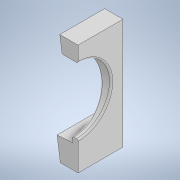
# Autodesk Inventor part: exhastForGasVent02
Saved by Autodesk Inventor 2021.1 (Build 251245000, 245)
## iProperties
Created: 2020-08-27
Part Number: exhastForGasVent02
Material: Generic
Document SubType Name: Modeling
Designer: robst
Density: 1 g/cm^3
Appearance: Default
Author: robst
Autodesk Inventor part; units mm, degrees
ref_plane "YZ Plane" through (0, 0, 0) normal (1, 0, 0) x (0, 1, 0)
ref_plane "XZ Plane" through (0, 0, 0) normal (0, 1, 0) x (-1, 0, 0)
ref_plane "XY Plane" through (0, 0, 0) normal (0, 0, 1) x (1, 0, 0)
sketch "Sketch6" plane through (0, 0, 0) normal (0, 0, 1) x (1, 0, 0)
  line L0 (0, 0) -> (0, 83.82)
  line L1 (0, 83.82) -> (-17.653, 83.82)
  line L2 (-17.653, 83.82) -> (-5.08, 0)
  line L3 (0, 0) -> (0, -22.86)
  line L4 (0, -22.86) -> (-17.091, -22.86)
  line L5 (-23.2881, 0) -> (-5.08, 0) construction
  line L6 (-5.08, 0) -> (-20.32, -1.3333)
  line L7 (-20.32, -1.3333) -> (-17.091, -22.86)
  dimension "d31" = 83.82
  dimension "d32" = 17.653
  dimension "d33" = 22.86
  dimension "d35" = 5
  dimension "d36" = 0
  dimension "d37" = 5.08
  dimension "d47" = 20.32
  constraints: 16 end point, 2 parallel, 2 perpendicular, 2 vertical
  measures "d31" distance of L0.start L0.end
  measures "d32" distance of L0.end L1.end
  measures "d33" distance of L0.start L3.end
  measures "d35" angle of L6 L5
  measures "d36" vertical distance of L2.end L0.start
  measures "d37" distance of L2.end L0.start
  measures "d47" distance from line of L6.end L3
extrude "Extrusion7" add sketch "Sketch6" along normal mid plane 86.36
sketch "Sketch7" plane through (0, -22.86, 43.18) normal (1, 0, 0) x (0, 0, -1)
  line L0 (86.36, 22.86) -> (0, 22.86) projected
  line L1 (0, 106.68) -> (86.36, 106.68) construction
  line L2 (43.18, 106.68) -> (43.18, 22.86) construction
  circle A0 centre (43.18, 59.69) radius 31.75
  dimension "d40" = 63.5
  dimension "d41" = 5.08
  constraints: 2 end point, 1 centre point, 1 midpoint, 1 perpendicular, 1 point on line
  measures "d40" diameter of A0
  measures "d41" distance edge to line of A0 L0
extrude "Extrusion8" cut sketch "Sketch7" against normal through all
sketch "Sketch11" plane through (-17.091, -22.86, -43.18) normal (-0.9889364, -0.1483405, 0) x (0, 0, 1)
  line L0 (43.18, 20.0718) -> (43.18, 0) construction
  line L1 (0, 0) -> (86.36, 0) construction
  line L2 (43.18, 10.0359) -> (86.36, 10.0359) construction
  spline S0 degree 2 poles (51.7003, 11.2824) (51.4336, 11.1738) (50.5806, 10.9663) (50.1656, 10.9663) knots 0 0 0 1 2 2 2
  spline S1 degree 2 poles (50.1656, 10.9663) (49.2073, 10.9663) (48.071, 12.0728) (48.071, 13.0872) knots 0 0 0 1 2 2 2
  spline S2 degree 2 poles (48.071, 13.0872) (48.071, 14.0423) (49.2073, 15.1949) (50.1953, 15.1949) knots 0 0 0 1 2 2 2
  spline S3 degree 2 poles (50.1953, 15.1949) (50.7057, 15.1949) (51.3446, 15.0006) (51.6839, 14.836) knots 0 0 0 1 2 2 2
  line L3 (51.6839, 14.836) -> (51.6839, 13.8809)
  line L4 (51.6839, 13.8809) -> (51.5916, 13.8809)
  spline S4 degree 2 poles (51.5916, 13.8809) (51.5192, 13.9369) (51.2425, 14.1509) (51.1108, 14.2234) knots 0 0 0 1 2 2 2
  spline S5 degree 2 poles (51.1108, 14.2234) (50.9593, 14.3123) (50.5575, 14.4375) (50.3336, 14.4375) knots 0 0 0 1 2 2 2
  spline S6 degree 2 poles (50.3336, 14.4375) (50.0734, 14.4375) (49.642, 14.2728) (49.474, 14.1048) knots 0 0 0 1 2 2 2
  spline S7 degree 2 poles (49.474, 14.1048) (49.3126, 13.9402) (49.1249, 13.4363) (49.1249, 13.1037) knots 0 0 0 1 2 2 2
  spline S8 degree 2 poles (49.1249, 13.1037) (49.1249, 12.3923) (49.8396, 11.7139) (50.4554, 11.7139) knots 0 0 0 1 2 2 2
  spline S9 degree 2 poles (50.4554, 11.7139) (50.5114, 11.7139) (50.6563, 11.7205) (50.7123, 11.7237) knots 0 0 0 1 2 2 2
  line L5 (50.7123, 11.7237) -> (50.7123, 12.524)
  line L6 (50.7123, 12.524) -> (49.9252, 12.524)
  line L7 (49.9252, 12.524) -> (49.9252, 13.2848)
  line L8 (49.9252, 13.2848) -> (51.7003, 13.2848)
  line L9 (51.7003, 13.2848) -> (51.7003, 11.2824)
  spline S10 degree 2 poles (54.1045, 11.3779) (54.0057, 11.2956) (53.8509, 11.1639) (53.7191, 11.098) knots 0 0 0 1 2 2 2
  spline S11 degree 2 poles (53.7191, 11.098) (53.5907, 11.0354) (53.347, 10.9696) (53.1296, 10.9696) knots 0 0 0 1 2 2 2
  spline S12 degree 2 poles (53.1296, 10.9696) (52.7213, 10.9696) (52.1844, 11.5163) (52.1844, 11.9312) knots 0 0 0 1 2 2 2
  spline S13 degree 2 poles (52.1844, 11.9312) (52.1844, 12.2704) (52.4578, 12.692) (52.7147, 12.8138) knots 0 0 0 1 2 2 2
  spline S14 degree 2 poles (52.7147, 12.8138) (52.9748, 12.939) (53.6961, 13.0378) (54.1111, 13.0641) knots 0 0 0 1 2 2 2
  line L10 (54.1111, 13.0641) -> (54.1111, 13.0806)
  spline S15 degree 2 poles (54.1111, 13.0806) (54.1111, 13.3342) (53.7356, 13.5285) (53.3602, 13.5285) knots 0 0 0 1 2 2 2
  spline S16 degree 2 poles (53.3602, 13.5285) (53.1922, 13.5285) (52.7377, 13.4066) (52.5237, 13.3111) knots 0 0 0 1 2 2 2
  line L11 (52.5237, 13.3111) -> (52.4413, 13.3111)
  line L12 (52.4413, 13.3111) -> (52.4413, 14.0521)
  spline S17 degree 2 poles (52.4413, 14.0521) (52.5829, 14.0917) (53.2153, 14.2036) (53.538, 14.2036) knots 0 0 0 1 2 2 2
  spline S18 degree 2 poles (53.538, 14.2036) (54.3284, 14.2036) (55.053, 13.6767) (55.053, 13.1366) knots 0 0 0 1 2 2 2
  line L13 (55.053, 13.1366) -> (55.053, 11.0519)
  line L14 (55.053, 11.0519) -> (54.1045, 11.0519)
  line L15 (54.1045, 11.0519) -> (54.1045, 11.3779)
  line L16 (54.1045, 11.8522) -> (54.1045, 12.4878)
  spline S19 degree 2 poles (54.1045, 12.4878) (53.8608, 12.4647) (53.5611, 12.4285) (53.4162, 12.3758) knots 0 0 0 1 2 2 2
  spline S20 degree 2 poles (53.4162, 12.3758) (53.2877, 12.333) (53.1494, 12.1552) (53.1494, 12.0103) knots 0 0 0 1 2 2 2
  spline S21 degree 2 poles (53.1494, 12.0103) (53.1494, 11.7962) (53.3832, 11.6348) (53.6105, 11.6348) knots 0 0 0 1 2 2 2
  spline S22 degree 2 poles (53.6105, 11.6348) (53.7356, 11.6348) (53.9991, 11.7501) (54.1045, 11.8522) knots 0 0 0 1 2 2 2
  spline S23 degree 2 poles (56.693, 10.9696) (56.3571, 10.9696) (55.7544, 11.1178) (55.5568, 11.2166) knots 0 0 0 1 2 2 2
  line L17 (55.5568, 11.2166) -> (55.5568, 12.0234)
  line L18 (55.5568, 12.0234) -> (55.6359, 12.0234)
  spline S24 degree 2 poles (55.6359, 12.0234) (55.705, 11.9707) (55.8796, 11.8456) (56.0344, 11.7764) knots 0 0 0 1 2 2 2
  spline S25 degree 2 poles (56.0344, 11.7764) (56.1694, 11.7139) (56.502, 11.6249) (56.6996, 11.6249) knots 0 0 0 1 2 2 2
  spline S26 degree 2 poles (56.6996, 11.6249) (56.9005, 11.6249) (57.2101, 11.7501) (57.2101, 11.8851) knots 0 0 0 1 2 2 2
  spline S27 degree 2 poles (57.2101, 11.8851) (57.2101, 11.9905) (57.0685, 12.1025) (56.8643, 12.1486) knots 0 0 0 1 2 2 2
  spline S28 degree 2 poles (56.8643, 12.1486) (56.7556, 12.1782) (56.423, 12.2408) (56.2946, 12.2803) knots 0 0 0 1 2 2 2
  spline S29 degree 2 poles (56.2946, 12.2803) (55.9323, 12.3923) (55.57, 12.8303) (55.57, 13.1893) knots 0 0 0 1 2 2 2
  spline S30 degree 2 poles (55.57, 13.1893) (55.57, 13.3935) (55.7577, 13.7557) (55.9422, 13.8974) knots 0 0 0 1 2 2 2
  spline S31 degree 2 poles (55.9422, 13.8974) (56.1233, 14.0357) (56.6601, 14.2003) (56.9993, 14.2003) knots 0 0 0 1 2 2 2
  spline S32 degree 2 poles (56.9993, 14.2003) (57.3221, 14.2003) (57.8622, 14.0719) (58.0466, 13.983) knots 0 0 0 1 2 2 2
  line L19 (58.0466, 13.983) -> (58.0466, 13.2058)
  line L20 (58.0466, 13.2058) -> (57.9709, 13.2058)
  spline S33 degree 2 poles (57.9709, 13.2058) (57.9215, 13.2453) (57.7074, 13.3737) (57.6086, 13.4198) knots 0 0 0 1 2 2 2
  spline S34 degree 2 poles (57.6086, 13.4198) (57.4867, 13.4725) (57.1903, 13.545) (57.0356, 13.545) knots 0 0 0 1 2 2 2
  spline S35 degree 2 poles (57.0356, 13.545) (56.8281, 13.545) (56.5416, 13.4034) (56.5416, 13.2881) knots 0 0 0 1 2 2 2
  spline S36 degree 2 poles (56.5416, 13.2881) (56.5416, 13.1827) (56.6832, 13.0641) (56.9203, 13.0049) knots 0 0 0 1 2 2 2
  spline S37 degree 2 poles (56.9203, 13.0049) (57.0421, 12.9752) (57.3616, 12.9192) (57.5098, 12.8698) knots 0 0 0 1 2 2 2
  spline S38 degree 2 poles (57.5098, 12.8698) (57.8391, 12.7644) (58.1816, 12.3528) (58.1816, 12.0103) knots 0 0 0 1 2 2 2
  spline S39 degree 2 poles (58.1816, 12.0103) (58.1816, 11.7962) (57.9807, 11.4043) (57.793, 11.2726) knots 0 0 0 1 2 2 2
  spline S40 degree 2 poles (57.793, 11.2726) (57.5987, 11.1276) (57.0652, 10.9696) (56.693, 10.9696) knots 0 0 0 1 2 2 2
  line L21 (63.7211, 15.1159) -> (62.3247, 11.0519)
  line L22 (62.3247, 11.0519) -> (61.2609, 11.0519)
  line L23 (61.2609, 11.0519) -> (59.8645, 15.1159)
  line L24 (59.8645, 15.1159) -> (60.9217, 15.1159)
  line L25 (60.9217, 15.1159) -> (61.8076, 12.3594)
  line L26 (61.8076, 12.3594) -> (62.6902, 15.1159)
  line L27 (62.6902, 15.1159) -> (63.7211, 15.1159)
  spline S41 degree 2 poles (65.7004, 10.9696) (64.8309, 10.9696) (63.9055, 11.7995) (63.9055, 12.5668) knots 0 0 0 1 2 2 2
  spline S42 degree 2 poles (63.9055, 12.5668) (63.9055, 13.3177) (64.7684, 14.2135) (65.5456, 14.2135) knots 0 0 0 1 2 2 2
  spline S43 degree 2 poles (65.5456, 14.2135) (66.2471, 14.2135) (66.9584, 13.4528) (66.9584, 12.748) knots 0 0 0 1 2 2 2
  line L28 (66.9584, 12.748) -> (66.9584, 12.4022)
  line L29 (66.9584, 12.4022) -> (64.8606, 12.4022)
  spline S44 degree 2 poles (64.8606, 12.4022) (64.8737, 12.1881) (65.0285, 11.9049) (65.1537, 11.8193) knots 0 0 0 1 2 2 2
  spline S45 degree 2 poles (65.1537, 11.8193) (65.2755, 11.7336) (65.6049, 11.6612) (65.7992, 11.6612) knots 0 0 0 1 2 2 2
  spline S46 degree 2 poles (65.7992, 11.6612) (65.9638, 11.6612) (66.2866, 11.7336) (66.4216, 11.7962) knots 0 0 0 1 2 2 2
  spline S47 degree 2 poles (66.4216, 11.7962) (66.5402, 11.8456) (66.7378, 11.9675) (66.8004, 12.0136) knots 0 0 0 1 2 2 2
  line L30 (66.8004, 12.0136) -> (66.9024, 12.0136)
  line L31 (66.9024, 12.0136) -> (66.9024, 11.2232)
  spline S48 degree 2 poles (66.9024, 11.2232) (66.7839, 11.177) (66.5929, 11.098) (66.4216, 11.0585) knots 0 0 0 1 2 2 2
  spline S49 degree 2 poles (66.4216, 11.0585) (66.2668, 11.0157) (65.9375, 10.9696) (65.7004, 10.9696) knots 0 0 0 1 2 2 2
  spline S50 degree 2 poles (66.0165, 12.9785) (66.0099, 13.2815) (65.7432, 13.601) (65.4698, 13.601) knots 0 0 0 1 2 2 2
  spline S51 degree 2 poles (65.4698, 13.601) (65.1899, 13.601) (64.8737, 13.265) (64.8573, 12.9785) knots 0 0 0 1 2 2 2
  line L32 (64.8573, 12.9785) -> (66.0165, 12.9785)
  line L33 (70.3177, 11.0519) -> (69.356, 11.0519)
  line L34 (69.356, 11.0519) -> (69.356, 12.5701)
  spline S52 degree 2 poles (69.356, 12.5701) (69.356, 12.7579) (69.3264, 13.1267) (69.2868, 13.2123) knots 0 0 0 1 2 2 2
  spline S53 degree 2 poles (69.2868, 13.2123) (69.2374, 13.3177) (69.053, 13.4066) (68.8949, 13.4066) knots 0 0 0 1 2 2 2
  spline S54 degree 2 poles (68.8949, 13.4066) (68.7797, 13.4066) (68.5392, 13.3177) (68.4042, 13.2222) knots 0 0 0 1 2 2 2
  line L35 (68.4042, 13.2222) -> (68.4042, 11.0519)
  line L36 (68.4042, 11.0519) -> (67.4491, 11.0519)
  line L37 (67.4491, 11.0519) -> (67.4491, 14.118)
  line L38 (67.4491, 14.118) -> (68.4042, 14.118)
  line L39 (68.4042, 14.118) -> (68.4042, 13.7788)
  spline S55 degree 2 poles (68.4042, 13.7788) (68.638, 13.9764) (69.0826, 14.2003) (69.3527, 14.2003) knots 0 0 0 1 2 2 2
  spline S56 degree 2 poles (69.3527, 14.2003) (69.8204, 14.2003) (70.3177, 13.6075) (70.3177, 13.0477) knots 0 0 0 1 2 2 2
  line L40 (70.3177, 13.0477) -> (70.3177, 11.0519)
  spline S57 degree 2 poles (72.1982, 10.9926) (71.6152, 10.9926) (71.0817, 11.4734) (71.0817, 12.0201) knots 0 0 0 1 2 2 2
  line L41 (71.0817, 12.0201) -> (71.0817, 13.4528)
  line L42 (71.0817, 13.4528) -> (70.7162, 13.4528)
  line L43 (70.7162, 13.4528) -> (70.7162, 14.118)
  line L44 (70.7162, 14.118) -> (71.0817, 14.118)
  line L45 (71.0817, 14.118) -> (71.0817, 14.994)
  line L46 (71.0817, 14.994) -> (72.0368, 14.994)
  line L47 (72.0368, 14.994) -> (72.0368, 14.118)
  line L48 (72.0368, 14.118) -> (72.9589, 14.118)
  line L49 (72.9589, 14.118) -> (72.9589, 13.4528)
  line L50 (72.9589, 13.4528) -> (72.0368, 13.4528)
  line L51 (72.0368, 13.4528) -> (72.0368, 12.3627)
  spline S58 degree 2 poles (72.0368, 12.3627) (72.0368, 12.2013) (72.0434, 11.9609) (72.0829, 11.8654) knots 0 0 0 1 2 2 2
  spline S59 degree 2 poles (72.0829, 11.8654) (72.1224, 11.7699) (72.3167, 11.6579) (72.5012, 11.6579) knots 0 0 0 1 2 2 2
  spline S60 degree 2 poles (72.5012, 11.6579) (72.5802, 11.6579) (72.8272, 11.7237) (72.8766, 11.7501) knots 0 0 0 1 2 2 2
  line L52 (72.8766, 11.7501) -> (72.9589, 11.7501)
  line L53 (72.9589, 11.7501) -> (72.9589, 11.0782)
  spline S61 degree 2 poles (72.9589, 11.0782) (72.8041, 11.0387) (72.455, 10.9926) (72.1982, 10.9926) knots 0 0 0 1 2 2 2
  spline S62 degree 2 poles (77.9648, 13.0839) (77.9648, 12.557) (77.7969, 11.7666) (77.6091, 11.4998) knots 0 0 0 1 2 2 2
  spline S63 degree 2 poles (77.6091, 11.4998) (77.4247, 11.2363) (76.8286, 10.9663) (76.4005, 10.9663) knots 0 0 0 1 2 2 2
  spline S64 degree 2 poles (76.4005, 10.9663) (75.9691, 10.9663) (75.3762, 11.2363) (75.1885, 11.5064) knots 0 0 0 1 2 2 2
  spline S65 degree 2 poles (75.1885, 11.5064) (75.0008, 11.7731) (74.8328, 12.557) (74.8328, 13.0839) knots 0 0 0 1 2 2 2
  spline S66 degree 2 poles (74.8328, 13.0839) (74.8328, 13.624) (75.0008, 14.3881) (75.1918, 14.6647) knots 0 0 0 1 2 2 2
  spline S67 degree 2 poles (75.1918, 14.6647) (75.3828, 14.9348) (75.9855, 15.1982) (76.4005, 15.1982) knots 0 0 0 1 2 2 2
  spline S68 degree 2 poles (76.4005, 15.1982) (76.8385, 15.1982) (77.4247, 14.9216) (77.6124, 14.6482) knots 0 0 0 1 2 2 2
  spline S69 degree 2 poles (77.6124, 14.6482) (77.7969, 14.3815) (77.9648, 13.5944) (77.9648, 13.0839) knots 0 0 0 1 2 2 2
  spline S70 degree 2 poles (76.9406, 13.0839) (76.9406, 13.8381) (76.6936, 14.4473) (76.4005, 14.4473) knots 0 0 0 1 2 2 2
  spline S71 degree 2 poles (76.4005, 14.4473) (76.1074, 14.4473) (75.8571, 13.8381) (75.8571, 13.0806) knots 0 0 0 1 2 2 2
  spline S72 degree 2 poles (75.8571, 13.0806) (75.8571, 12.3363) (76.1074, 11.7172) (76.4005, 11.7172) knots 0 0 0 1 2 2 2
  spline S73 degree 2 poles (76.4005, 11.7172) (76.6903, 11.7172) (76.9406, 12.3363) (76.9406, 13.0839) knots 0 0 0 1 2 2 2
  line L54 (81.5776, 11.0519) -> (78.5906, 11.0519)
  line L55 (78.5906, 11.0519) -> (78.5906, 11.7139)
  spline S74 degree 2 poles (78.5906, 11.7139) (78.9693, 12.0169) (79.5753, 12.5504) (79.8025, 12.7908) knots 0 0 0 1 2 2 2
  spline S75 degree 2 poles (79.8025, 12.7908) (80.1022, 13.1037) (80.369, 13.5812) (80.369, 13.8315) knots 0 0 0 1 2 2 2
  spline S76 degree 2 poles (80.369, 13.8315) (80.369, 14.1147) (80.0298, 14.4177) (79.7268, 14.4177) knots 0 0 0 1 2 2 2
  spline S77 degree 2 poles (79.7268, 14.4177) (79.572, 14.4177) (79.2953, 14.342) (79.1537, 14.2827) knots 0 0 0 1 2 2 2
  spline S78 degree 2 poles (79.1537, 14.2827) (79.0154, 14.2201) (78.8178, 14.0884) (78.7684, 14.0554) knots 0 0 0 1 2 2 2
  line L56 (78.7684, 14.0554) -> (78.6894, 14.0554)
  line L57 (78.6894, 14.0554) -> (78.6894, 14.9414)
  spline S79 degree 2 poles (78.6894, 14.9414) (78.8606, 15.0237) (79.5917, 15.1949) (79.931, 15.1949) knots 0 0 0 1 2 2 2
  spline S80 degree 2 poles (79.931, 15.1949) (80.6555, 15.1949) (81.3998, 14.5494) (81.3998, 13.9665) knots 0 0 0 1 2 2 2
  spline S81 degree 2 poles (81.3998, 13.9665) (81.3998, 13.6075) (81.0606, 12.9159) (80.6687, 12.5207) knots 0 0 0 1 2 2 2
  spline S82 degree 2 poles (80.6687, 12.5207) (80.4217, 12.277) (79.9573, 11.8983) (79.8552, 11.8193) knots 0 0 0 1 2 2 2
  line L58 (79.8552, 11.8193) -> (81.5776, 11.8193)
  line L59 (81.5776, 11.8193) -> (81.5776, 11.0519)
  spline S83 degree 2 poles (54.0073, 7.0249) (54.0073, 6.7416) (53.8262, 6.2279) (53.6582, 6.0566) knots 0 0 0 1 2 2 2
  spline S84 degree 2 poles (53.6582, 6.0566) (53.5561, 5.9479) (53.3058, 5.7701) (53.1576, 5.7075) knots 0 0 0 1 2 2 2
  spline S85 degree 2 poles (53.1576, 5.7075) (53.0061, 5.6449) (52.6537, 5.5725) (52.4364, 5.5725) knots 0 0 0 1 2 2 2
  line L60 (52.4364, 5.5725) -> (51.9029, 5.5725)
  line L61 (51.9029, 5.5725) -> (51.9029, 4.242)
  line L62 (51.9029, 4.242) -> (50.8819, 4.242)
  line L63 (50.8819, 4.242) -> (50.8819, 8.306)
  line L64 (50.8819, 8.306) -> (52.4594, 8.306)
  spline S86 degree 2 poles (52.4594, 8.306) (52.8085, 8.306) (53.319, 8.1775) (53.5265, 8.0392) knots 0 0 0 1 2 2 2
  spline S87 degree 2 poles (53.5265, 8.0392) (53.757, 7.8844) (54.0073, 7.3772) (54.0073, 7.0249) knots 0 0 0 1 2 2 2
  spline S88 degree 2 poles (52.96, 6.9985) (52.96, 7.1731) (52.7954, 7.4201) (52.6834, 7.4662) knots 0 0 0 1 2 2 2
  spline S89 degree 2 poles (52.6834, 7.4662) (52.5385, 7.5287) (52.275, 7.5485) (52.0478, 7.5485) knots 0 0 0 1 2 2 2
  line L65 (52.0478, 7.5485) -> (51.9029, 7.5485)
  line L66 (51.9029, 7.5485) -> (51.9029, 6.33)
  line L67 (51.9029, 6.33) -> (51.9753, 6.33)
  spline S90 degree 2 poles (51.9753, 6.33) (52.1169, 6.33) (52.3738, 6.3365) (52.4693, 6.353) knots 0 0 0 1 2 2 2
  spline S91 degree 2 poles (52.4693, 6.353) (52.5517, 6.3662) (52.7328, 6.4452) (52.7822, 6.4946) knots 0 0 0 1 2 2 2
  spline S92 degree 2 poles (52.7822, 6.4946) (52.8876, 6.5934) (52.96, 6.8141) (52.96, 6.9985) knots 0 0 0 1 2 2 2
  line L68 (56.5564, 6.4024) -> (56.4773, 6.4024)
  spline S93 degree 2 poles (56.4773, 6.4024) (56.4213, 6.4222) (56.2139, 6.4419) (56.0887, 6.4419) knots 0 0 0 1 2 2 2
  spline S94 degree 2 poles (56.0887, 6.4419) (55.9405, 6.4419) (55.6079, 6.353) (55.4531, 6.2937) knots 0 0 0 1 2 2 2
  line L69 (55.4531, 6.2937) -> (55.4531, 4.242)
  line L70 (55.4531, 4.242) -> (54.498, 4.242)
  line L71 (54.498, 4.242) -> (54.498, 7.3081)
  line L72 (54.498, 7.3081) -> (55.4531, 7.3081)
  line L73 (55.4531, 7.3081) -> (55.4531, 6.8668)
  spline S95 degree 2 poles (55.4531, 6.8668) (55.519, 6.9261) (55.7495, 7.1105) (55.845, 7.1665) knots 0 0 0 1 2 2 2
  spline S96 degree 2 poles (55.845, 7.1665) (55.9504, 7.229) (56.227, 7.318) (56.3489, 7.318) knots 0 0 0 1 2 2 2
  spline S97 degree 2 poles (56.3489, 7.318) (56.395, 7.318) (56.5103, 7.3114) (56.5564, 7.3081) knots 0 0 0 1 2 2 2
  line L74 (56.5564, 7.3081) -> (56.5564, 6.4024)
  line L75 (57.877, 4.242) -> (56.9219, 4.242)
  line L76 (56.9219, 4.242) -> (56.9219, 7.3081)
  line L77 (56.9219, 7.3081) -> (57.877, 7.3081)
  line L78 (57.877, 7.3081) -> (57.877, 4.242)
  line L79 (57.9066, 7.7461) -> (56.8956, 7.7461)
  line L80 (56.8956, 7.7461) -> (56.8956, 8.4904)
  line L81 (56.8956, 8.4904) -> (57.9066, 8.4904)
  line L82 (57.9066, 8.4904) -> (57.9066, 7.7461)
  line L83 (61.4766, 4.242) -> (60.515, 4.242)
  line L84 (60.515, 4.242) -> (60.515, 5.7602)
  spline S98 degree 2 poles (60.515, 5.7602) (60.515, 5.9479) (60.4853, 6.3168) (60.4458, 6.4024) knots 0 0 0 1 2 2 2
  spline S99 degree 2 poles (60.4458, 6.4024) (60.3964, 6.5078) (60.212, 6.5967) (60.0539, 6.5967) knots 0 0 0 1 2 2 2
  spline S100 degree 2 poles (60.0539, 6.5967) (59.9386, 6.5967) (59.6982, 6.5078) (59.5632, 6.4123) knots 0 0 0 1 2 2 2
  line L85 (59.5632, 6.4123) -> (59.5632, 4.242)
  line L86 (59.5632, 4.242) -> (58.6081, 4.242)
  line L87 (58.6081, 4.242) -> (58.6081, 7.3081)
  line L88 (58.6081, 7.3081) -> (59.5632, 7.3081)
  line L89 (59.5632, 7.3081) -> (59.5632, 6.9689)
  spline S101 degree 2 poles (59.5632, 6.9689) (59.797, 7.1665) (60.2416, 7.3904) (60.5117, 7.3904) knots 0 0 0 1 2 2 2
  spline S102 degree 2 poles (60.5117, 7.3904) (60.9793, 7.3904) (61.4766, 6.7976) (61.4766, 6.2377) knots 0 0 0 1 2 2 2
  line L90 (61.4766, 6.2377) -> (61.4766, 4.242)
  spline S103 degree 2 poles (63.3572, 4.1827) (62.7742, 4.1827) (62.2407, 4.6635) (62.2407, 5.2102) knots 0 0 0 1 2 2 2
  line L91 (62.2407, 5.2102) -> (62.2407, 6.6428)
  line L92 (62.2407, 6.6428) -> (61.8751, 6.6428)
  line L93 (61.8751, 6.6428) -> (61.8751, 7.3081)
  line L94 (61.8751, 7.3081) -> (62.2407, 7.3081)
  line L95 (62.2407, 7.3081) -> (62.2407, 8.1841)
  line L96 (62.2407, 8.1841) -> (63.1958, 8.1841)
  line L97 (63.1958, 8.1841) -> (63.1958, 7.3081)
  line L98 (63.1958, 7.3081) -> (64.1179, 7.3081)
  line L99 (64.1179, 7.3081) -> (64.1179, 6.6428)
  line L100 (64.1179, 6.6428) -> (63.1958, 6.6428)
  line L101 (63.1958, 6.6428) -> (63.1958, 5.5527)
  spline S104 degree 2 poles (63.1958, 5.5527) (63.1958, 5.3914) (63.2024, 5.1509) (63.2419, 5.0554) knots 0 0 0 1 2 2 2
  spline S105 degree 2 poles (63.2419, 5.0554) (63.2814, 4.9599) (63.4757, 4.848) (63.6601, 4.848) knots 0 0 0 1 2 2 2
  spline S106 degree 2 poles (63.6601, 4.848) (63.7392, 4.848) (63.9862, 4.9138) (64.0356, 4.9402) knots 0 0 0 1 2 2 2
  line L102 (64.0356, 4.9402) -> (64.1179, 4.9402)
  line L103 (64.1179, 4.9402) -> (64.1179, 4.2683)
  spline S107 degree 2 poles (64.1179, 4.2683) (63.9631, 4.2288) (63.614, 4.1827) (63.3572, 4.1827) knots 0 0 0 1 2 2 2
  line L104 (69.5915, 8.306) -> (68.1951, 4.242)
  line L105 (68.1951, 4.242) -> (67.1313, 4.242)
  line L106 (67.1313, 4.242) -> (65.735, 8.306)
  line L107 (65.735, 8.306) -> (66.7921, 8.306)
  line L108 (66.7921, 8.306) -> (67.678, 5.5494)
  line L109 (67.678, 5.5494) -> (68.5607, 8.306)
  line L110 (68.5607, 8.306) -> (69.5915, 8.306)
  line L111 (71.742, 5.6581) -> (69.934, 5.6581)
  line L112 (69.934, 5.6581) -> (69.934, 6.4156)
  line L113 (69.934, 6.4156) -> (71.742, 6.4156)
  line L114 (71.742, 6.4156) -> (71.742, 5.6581)
  spline S108 degree 2 poles (75.3911, 6.274) (75.3911, 5.747) (75.2231, 4.9566) (75.0354, 4.6899) knots 0 0 0 1 2 2 2
  spline S109 degree 2 poles (75.0354, 4.6899) (74.851, 4.4264) (74.2549, 4.1563) (73.8267, 4.1563) knots 0 0 0 1 2 2 2
  spline S110 degree 2 poles (73.8267, 4.1563) (73.3953, 4.1563) (72.8025, 4.4264) (72.6148, 4.6965) knots 0 0 0 1 2 2 2
  spline S111 degree 2 poles (72.6148, 4.6965) (72.4271, 4.9632) (72.2591, 5.747) (72.2591, 6.274) knots 0 0 0 1 2 2 2
  spline S112 degree 2 poles (72.2591, 6.274) (72.2591, 6.8141) (72.4271, 7.5781) (72.6181, 7.8548) knots 0 0 0 1 2 2 2
  spline S113 degree 2 poles (72.6181, 7.8548) (72.8091, 8.1248) (73.4118, 8.3883) (73.8267, 8.3883) knots 0 0 0 1 2 2 2
  spline S114 degree 2 poles (73.8267, 8.3883) (74.2647, 8.3883) (74.851, 8.1117) (75.0387, 7.8383) knots 0 0 0 1 2 2 2
  spline S115 degree 2 poles (75.0387, 7.8383) (75.2231, 7.5716) (75.3911, 6.7844) (75.3911, 6.274) knots 0 0 0 1 2 2 2
  spline S116 degree 2 poles (74.3668, 6.274) (74.3668, 7.0282) (74.1198, 7.6374) (73.8267, 7.6374) knots 0 0 0 1 2 2 2
  spline S117 degree 2 poles (73.8267, 7.6374) (73.5336, 7.6374) (73.2833, 7.0282) (73.2833, 6.2707) knots 0 0 0 1 2 2 2
  spline S118 degree 2 poles (73.2833, 6.2707) (73.2833, 5.5264) (73.5336, 4.9072) (73.8267, 4.9072) knots 0 0 0 1 2 2 2
  spline S119 degree 2 poles (73.8267, 4.9072) (74.1165, 4.9072) (74.3668, 5.5264) (74.3668, 6.274) knots 0 0 0 1 2 2 2
  line L115 (79.0039, 4.242) -> (76.0168, 4.242)
  line L116 (76.0168, 4.242) -> (76.0168, 4.9039)
  spline S120 degree 2 poles (76.0168, 4.9039) (76.3955, 5.2069) (77.0015, 5.7405) (77.2288, 5.9809) knots 0 0 0 1 2 2 2
  spline S121 degree 2 poles (77.2288, 5.9809) (77.5285, 6.2937) (77.7952, 6.7713) (77.7952, 7.0216) knots 0 0 0 1 2 2 2
  spline S122 degree 2 poles (77.7952, 7.0216) (77.7952, 7.3048) (77.456, 7.6078) (77.153, 7.6078) knots 0 0 0 1 2 2 2
  spline S123 degree 2 poles (77.153, 7.6078) (76.9982, 7.6078) (76.7216, 7.532) (76.58, 7.4728) knots 0 0 0 1 2 2 2
  spline S124 degree 2 poles (76.58, 7.4728) (76.4416, 7.4102) (76.244, 7.2784) (76.1946, 7.2455) knots 0 0 0 1 2 2 2
  line L117 (76.1946, 7.2455) -> (76.1156, 7.2455)
  line L118 (76.1156, 7.2455) -> (76.1156, 8.1314)
  spline S125 degree 2 poles (76.1156, 8.1314) (76.2869, 8.2138) (77.018, 8.385) (77.3572, 8.385) knots 0 0 0 1 2 2 2
  spline S126 degree 2 poles (77.3572, 8.385) (78.0817, 8.385) (78.826, 7.7395) (78.826, 7.1566) knots 0 0 0 1 2 2 2
  spline S127 degree 2 poles (78.826, 7.1566) (78.826, 6.7976) (78.4868, 6.106) (78.0949, 5.7108) knots 0 0 0 1 2 2 2
  spline S128 degree 2 poles (78.0949, 5.7108) (77.8479, 5.4671) (77.3835, 5.0884) (77.2815, 5.0093) knots 0 0 0 1 2 2 2
  line L119 (77.2815, 5.0093) -> (79.0039, 5.0093)
  line L120 (79.0039, 5.0093) -> (79.0039, 4.242)
  constraints: 4 end point, 2 horizontal, 2 midpoint
extrude "Extrusion11" cut sketch "Sketch11" against normal blind 1.27
fillet "Fillet1" radius 1.5875 2 edges at (0, 36.83, 31.75) (-10.6045, 36.83, 31.75)
sketch "Sketch12" plane through (-17.091, -22.86, -43.18) normal (-0.9889364, -0.1483405, 0) x (0, 0, 1)
  line L0 (43.18, 20.0718) -> (43.18, 0) construction
  line L1 (0, 0) -> (86.36, 0) construction
  line L2 (43.18, 10.0359) -> (0, 10.0359) construction
  line L3 (0, 0) -> (0, 21.7675) construction
  spline S0 degree 2 poles (8.6982, 10.9729) (8.2667, 10.9729) (7.5521, 11.2363) (7.2952, 11.5031) knots 0 0 0 1 2 2 2
  spline S1 degree 2 poles (7.2952, 11.5031) (7.0383, 11.7731) (6.765, 12.5701) (6.765, 13.0872) knots 0 0 0 1 2 2 2
  spline S2 degree 2 poles (6.765, 13.0872) (6.765, 13.5779) (7.0416, 14.3551) (7.2985, 14.6318) knots 0 0 0 1 2 2 2
  spline S3 degree 2 poles (7.2985, 14.6318) (7.5455, 14.8985) (8.27, 15.1884) (8.7015, 15.1884) knots 0 0 0 1 2 2 2
  spline S4 degree 2 poles (8.7015, 15.1884) (8.9089, 15.1884) (9.2844, 15.1291) (9.4556, 15.0764) knots 0 0 0 1 2 2 2
  spline S5 degree 2 poles (9.4556, 15.0764) (9.594, 15.0369) (9.9299, 14.892) (10.032, 14.8393) knots 0 0 0 1 2 2 2
  line L4 (10.032, 14.8393) -> (10.032, 14.1872)
  line L5 (10.032, 14.1872) -> (9.9859, 14.1872)
  spline S6 degree 2 poles (9.9859, 14.1872) (9.8838, 14.2761) (9.6697, 14.4375) (9.4721, 14.5297) knots 0 0 0 1 2 2 2
  spline S7 degree 2 poles (9.4721, 14.5297) (9.3074, 14.612) (8.8826, 14.7207) (8.6389, 14.7207) knots 0 0 0 1 2 2 2
  spline S8 degree 2 poles (8.6389, 14.7207) (8.0527, 14.7207) (7.3281, 13.8381) (7.3281, 13.1037) knots 0 0 0 1 2 2 2
  spline S9 degree 2 poles (7.3281, 13.1037) (7.3281, 12.6953) (7.5191, 12.0827) (7.7003, 11.8719) knots 0 0 0 1 2 2 2
  spline S10 degree 2 poles (7.7003, 11.8719) (7.8748, 11.6612) (8.3688, 11.4405) (8.6784, 11.4405) knots 0 0 0 1 2 2 2
  spline S11 degree 2 poles (8.6784, 11.4405) (8.9056, 11.4405) (9.3601, 11.5064) (9.5149, 11.5722) knots 0 0 0 1 2 2 2
  line L6 (9.5149, 11.5722) -> (9.5149, 12.6228)
  line L7 (9.5149, 12.6228) -> (8.573, 12.6228)
  line L8 (8.573, 12.6228) -> (8.573, 13.0971)
  line L9 (8.573, 13.0971) -> (10.0484, 13.0971)
  line L10 (10.0484, 13.0971) -> (10.0484, 11.322)
  spline S12 degree 2 poles (10.0484, 11.322) (9.9463, 11.2758) (9.5972, 11.1342) (9.449, 11.0914) knots 0 0 0 1 2 2 2
  spline S13 degree 2 poles (9.449, 11.0914) (9.2482, 11.0321) (8.9254, 10.9729) (8.6982, 10.9729) knots 0 0 0 1 2 2 2
  spline S14 degree 2 poles (12.3867, 11.3746) (12.3241, 11.3285) (12.1134, 11.1639) (12.0146, 11.1145) knots 0 0 0 1 2 2 2
  spline S15 degree 2 poles (12.0146, 11.1145) (11.8795, 11.042) (11.626, 10.9663) (11.3954, 10.9663) knots 0 0 0 1 2 2 2
  spline S16 degree 2 poles (11.3954, 10.9663) (11.2077, 10.9663) (10.8685, 11.1079) (10.74, 11.2363) knots 0 0 0 1 2 2 2
  spline S17 degree 2 poles (10.74, 11.2363) (10.6182, 11.3615) (10.47, 11.7303) (10.47, 11.9345) knots 0 0 0 1 2 2 2
  spline S18 degree 2 poles (10.47, 11.9345) (10.47, 12.2507) (10.7367, 12.6986) (11.0266, 12.827) knots 0 0 0 1 2 2 2
  spline S19 degree 2 poles (11.0266, 12.827) (11.2834, 12.9456) (11.9816, 13.0345) (12.3867, 13.0576) knots 0 0 0 1 2 2 2
  line L11 (12.3867, 13.0576) -> (12.3867, 13.1564)
  spline S20 degree 2 poles (12.3867, 13.1564) (12.3867, 13.3342) (12.278, 13.5548) (12.1792, 13.6174) knots 0 0 0 1 2 2 2
  spline S21 degree 2 poles (12.1792, 13.6174) (12.0804, 13.68) (11.7972, 13.7195) (11.6457, 13.7195) knots 0 0 0 1 2 2 2
  spline S22 degree 2 poles (11.6457, 13.7195) (11.4679, 13.7195) (10.987, 13.6141) (10.7466, 13.512) knots 0 0 0 1 2 2 2
  line L12 (10.7466, 13.512) -> (10.717, 13.512)
  line L13 (10.717, 13.512) -> (10.717, 14.0357)
  spline S23 degree 2 poles (10.717, 14.0357) (10.8586, 14.0752) (11.3888, 14.174) (11.649, 14.174) knots 0 0 0 1 2 2 2
  spline S24 degree 2 poles (11.649, 14.174) (11.9652, 14.174) (12.3966, 14.0752) (12.5679, 13.9468) knots 0 0 0 1 2 2 2
  spline S25 degree 2 poles (12.5679, 13.9468) (12.7358, 13.8216) (12.9005, 13.4231) (12.9005, 13.1366) knots 0 0 0 1 2 2 2
  line L14 (12.9005, 13.1366) -> (12.9005, 11.0519)
  line L15 (12.9005, 11.0519) -> (12.3867, 11.0519)
  line L16 (12.3867, 11.0519) -> (12.3867, 11.3746)
  line L17 (12.3867, 11.8028) -> (12.3867, 12.6492)
  spline S26 degree 2 poles (12.3867, 12.6492) (12.2023, 12.6327) (11.6457, 12.5767) (11.4712, 12.524) knots 0 0 0 1 2 2 2
  spline S27 degree 2 poles (11.4712, 12.524) (11.267, 12.4615) (11.0002, 12.2013) (11.0002, 11.9707) knots 0 0 0 1 2 2 2
  spline S28 degree 2 poles (11.0002, 11.9707) (11.0002, 11.7073) (11.2966, 11.4405) (11.5798, 11.4405) knots 0 0 0 1 2 2 2
  spline S29 degree 2 poles (11.5798, 11.4405) (11.8203, 11.4405) (12.2155, 11.648) (12.3867, 11.8028) knots 0 0 0 1 2 2 2
  spline S30 degree 2 poles (14.4451, 10.9794) (14.1388, 10.9794) (13.6086, 11.1441) (13.434, 11.2363) knots 0 0 0 1 2 2 2
  line L18 (13.434, 11.2363) -> (13.434, 11.8127)
  line L19 (13.434, 11.8127) -> (13.4604, 11.8127)
  spline S31 degree 2 poles (13.4604, 11.8127) (13.5262, 11.76) (13.7041, 11.6348) (13.8523, 11.5657) knots 0 0 0 1 2 2 2
  spline S32 degree 2 poles (13.8523, 11.5657) (13.9807, 11.5031) (14.2969, 11.4109) (14.4648, 11.4109) knots 0 0 0 1 2 2 2
  spline S33 degree 2 poles (14.4648, 11.4109) (14.5867, 11.4109) (14.8666, 11.4669) (14.9325, 11.513) knots 0 0 0 1 2 2 2
  spline S34 degree 2 poles (14.9325, 11.513) (15.028, 11.5755) (15.1136, 11.7172) (15.1136, 11.8621) knots 0 0 0 1 2 2 2
  spline S35 degree 2 poles (15.1136, 11.8621) (15.1136, 12.0432) (14.916, 12.2309) (14.6624, 12.2935) knots 0 0 0 1 2 2 2
  spline S36 degree 2 poles (14.6624, 12.2935) (14.5636, 12.3165) (14.2475, 12.3824) (14.1124, 12.4186) knots 0 0 0 1 2 2 2
  spline S37 degree 2 poles (14.1124, 12.4186) (13.7633, 12.5207) (13.4472, 12.9423) (13.4472, 13.242) knots 0 0 0 1 2 2 2
  spline S38 degree 2 poles (13.4472, 13.242) (13.4472, 13.6569) (14.0696, 14.174) (14.5834, 14.174) knots 0 0 0 1 2 2 2
  spline S39 degree 2 poles (14.5834, 14.174) (14.837, 14.174) (15.3507, 14.0489) (15.5253, 13.9533) knots 0 0 0 1 2 2 2
  line L20 (15.5253, 13.9533) -> (15.5253, 13.4034)
  line L21 (15.5253, 13.4034) -> (15.4989, 13.4034)
  spline S40 degree 2 poles (15.4989, 13.4034) (15.3013, 13.5614) (14.8205, 13.7426) (14.5735, 13.7426) knots 0 0 0 1 2 2 2
  spline S41 degree 2 poles (14.5735, 13.7426) (14.3199, 13.7426) (13.9708, 13.5285) (13.9708, 13.3144) knots 0 0 0 1 2 2 2
  spline S42 degree 2 poles (13.9708, 13.3144) (13.9708, 13.1201) (14.1783, 12.9324) (14.4088, 12.8731) knots 0 0 0 1 2 2 2
  spline S43 degree 2 poles (14.4088, 12.8731) (14.5208, 12.8435) (14.804, 12.7842) (14.9588, 12.748) knots 0 0 0 1 2 2 2
  spline S44 degree 2 poles (14.9588, 12.748) (15.2948, 12.6623) (15.6373, 12.2704) (15.6373, 11.9312) knots 0 0 0 1 2 2 2
  spline S45 degree 2 poles (15.6373, 11.9312) (15.6373, 11.7336) (15.4825, 11.3845) (15.331, 11.2561) knots 0 0 0 1 2 2 2
  spline S46 degree 2 poles (15.331, 11.2561) (15.1696, 11.1211) (14.7579, 10.9794) (14.4451, 10.9794) knots 0 0 0 1 2 2 2
  line L22 (20.8473, 15.1159) -> (19.4477, 11.0519)
  line L23 (19.4477, 11.0519) -> (18.8647, 11.0519)
  line L24 (18.8647, 11.0519) -> (17.4651, 15.1159)
  line L25 (17.4651, 15.1159) -> (18.0447, 15.1159)
  line L26 (18.0447, 15.1159) -> (19.171, 11.7402)
  line L27 (19.171, 11.7402) -> (20.2974, 15.1159)
  line L28 (20.2974, 15.1159) -> (20.8473, 15.1159)
  spline S47 degree 2 poles (22.5665, 10.9827) (21.8354, 10.9827) (21.0318, 11.8028) (21.0318, 12.5603) knots 0 0 0 1 2 2 2
  spline S48 degree 2 poles (21.0318, 12.5603) (21.0318, 13.3046) (21.8123, 14.1872) (22.4413, 14.1872) knots 0 0 0 1 2 2 2
  spline S49 degree 2 poles (22.4413, 14.1872) (22.7246, 14.1872) (23.1626, 14.0225) (23.324, 13.848) knots 0 0 0 1 2 2 2
  spline S50 degree 2 poles (23.324, 13.848) (23.4886, 13.6734) (23.6632, 13.1695) (23.6632, 12.804) knots 0 0 0 1 2 2 2
  line L29 (23.6632, 12.804) -> (23.6632, 12.524)
  line L30 (23.6632, 12.524) -> (21.5521, 12.524)
  spline S51 degree 2 poles (21.5521, 12.524) (21.5521, 11.9938) (22.0856, 11.4306) (22.5599, 11.4306) knots 0 0 0 1 2 2 2
  spline S52 degree 2 poles (22.5599, 11.4306) (22.7279, 11.4306) (23.0539, 11.5064) (23.1856, 11.5657) knots 0 0 0 1 2 2 2
  spline S53 degree 2 poles (23.1856, 11.5657) (23.324, 11.6315) (23.515, 11.7468) (23.5775, 11.7995) knots 0 0 0 1 2 2 2
  line L31 (23.5775, 11.7995) -> (23.6072, 11.7995)
  line L32 (23.6072, 11.7995) -> (23.6072, 11.2396)
  spline S54 degree 2 poles (23.6072, 11.2396) (23.5183, 11.2034) (23.2482, 11.098) (23.1428, 11.0684) knots 0 0 0 1 2 2 2
  spline S55 degree 2 poles (23.1428, 11.0684) (22.9946, 11.0256) (22.7509, 10.9827) (22.5665, 10.9827) knots 0 0 0 1 2 2 2
  spline S56 degree 2 poles (23.1626, 12.9159) (23.156, 13.1234) (23.0704, 13.4264) (22.988, 13.5285) knots 0 0 0 1 2 2 2
  spline S57 degree 2 poles (22.988, 13.5285) (22.8991, 13.6438) (22.6192, 13.7656) (22.4117, 13.7656) knots 0 0 0 1 2 2 2
  spline S58 degree 2 poles (22.4117, 13.7656) (22.2075, 13.7656) (21.921, 13.6438) (21.8024, 13.5252) knots 0 0 0 1 2 2 2
  spline S59 degree 2 poles (21.8024, 13.5252) (21.6872, 13.4034) (21.5686, 13.1102) (21.5521, 12.9159) knots 0 0 0 1 2 2 2
  line L33 (21.5521, 12.9159) -> (23.1626, 12.9159)
  line L34 (26.5778, 11.0519) -> (26.064, 11.0519)
  line L35 (26.064, 11.0519) -> (26.064, 12.7908)
  spline S60 degree 2 poles (26.064, 12.7908) (26.064, 13.0016) (26.0245, 13.3638) (25.9652, 13.4725) knots 0 0 0 1 2 2 2
  spline S61 degree 2 poles (25.9652, 13.4725) (25.9026, 13.5878) (25.6787, 13.6998) (25.4877, 13.6998) knots 0 0 0 1 2 2 2
  spline S62 degree 2 poles (25.4877, 13.6998) (25.2967, 13.6998) (24.8916, 13.4956) (24.6973, 13.3309) knots 0 0 0 1 2 2 2
  line L36 (24.6973, 13.3309) -> (24.6973, 11.0519)
  line L37 (24.6973, 11.0519) -> (24.1835, 11.0519)
  line L38 (24.1835, 11.0519) -> (24.1835, 14.1015)
  line L39 (24.1835, 14.1015) -> (24.6973, 14.1015)
  line L40 (24.6973, 14.1015) -> (24.6973, 13.7623)
  spline S63 degree 2 poles (24.6973, 13.7623) (24.9278, 13.9698) (25.3724, 14.1872) (25.6227, 14.1872) knots 0 0 0 1 2 2 2
  spline S64 degree 2 poles (25.6227, 14.1872) (26.0706, 14.1872) (26.5778, 13.5944) (26.5778, 13.0312) knots 0 0 0 1 2 2 2
  line L41 (26.5778, 13.0312) -> (26.5778, 11.0519)
  spline S65 degree 2 poles (28.2212, 10.9926) (27.8029, 10.9926) (27.332, 11.4702) (27.332, 11.9872) knots 0 0 0 1 2 2 2
  line L42 (27.332, 11.9872) -> (27.332, 13.6767)
  line L43 (27.332, 13.6767) -> (26.9862, 13.6767)
  line L44 (26.9862, 13.6767) -> (26.9862, 14.1015)
  line L45 (26.9862, 14.1015) -> (27.332, 14.1015)
  line L46 (27.332, 14.1015) -> (27.332, 14.9776)
  line L47 (27.332, 14.9776) -> (27.8457, 14.9776)
  line L48 (27.8457, 14.9776) -> (27.8457, 14.1015)
  line L49 (27.8457, 14.1015) -> (28.7909, 14.1015)
  line L50 (28.7909, 14.1015) -> (28.7909, 13.6767)
  line L51 (28.7909, 13.6767) -> (27.8457, 13.6767)
  line L52 (27.8457, 13.6767) -> (27.8457, 12.2243)
  spline S66 degree 2 poles (27.8457, 12.2243) (27.8457, 11.9938) (27.8622, 11.7402) (27.9182, 11.6315) knots 0 0 0 1 2 2 2
  spline S67 degree 2 poles (27.9182, 11.6315) (27.9643, 11.536) (28.1718, 11.4405) (28.3496, 11.4405) knots 0 0 0 1 2 2 2
  spline S68 degree 2 poles (28.3496, 11.4405) (28.4748, 11.4405) (28.7086, 11.5163) (28.7613, 11.5393) knots 0 0 0 1 2 2 2
  line L53 (28.7613, 11.5393) -> (28.7909, 11.5393)
  line L54 (28.7909, 11.5393) -> (28.7909, 11.0782)
  spline S69 degree 2 poles (28.7909, 11.0782) (28.646, 11.0387) (28.3496, 10.9926) (28.2212, 10.9926) knots 0 0 0 1 2 2 2
  spline S70 degree 2 poles (33.3687, 13.0839) (33.3687, 11.9905) (32.7331, 10.9663) (32.0711, 10.9663) knots 0 0 0 1 2 2 2
  spline S71 degree 2 poles (32.0711, 10.9663) (31.3993, 10.9663) (30.7702, 12.0103) (30.7702, 13.0806) knots 0 0 0 1 2 2 2
  spline S72 degree 2 poles (30.7702, 13.0806) (30.7702, 14.1806) (31.4058, 15.1982) (32.0711, 15.1982) knots 0 0 0 1 2 2 2
  spline S73 degree 2 poles (32.0711, 15.1982) (32.7397, 15.1982) (33.3687, 14.1444) (33.3687, 13.0839) knots 0 0 0 1 2 2 2
  spline S74 degree 2 poles (32.6705, 11.8456) (32.7495, 12.0465) (32.8154, 12.6656) (32.8154, 13.0839) knots 0 0 0 1 2 2 2
  spline S75 degree 2 poles (32.8154, 13.0839) (32.8154, 13.5022) (32.7495, 14.118) (32.6672, 14.3255) knots 0 0 0 1 2 2 2
  spline S76 degree 2 poles (32.6672, 14.3255) (32.5849, 14.533) (32.2983, 14.747) (32.0711, 14.747) knots 0 0 0 1 2 2 2
  spline S77 degree 2 poles (32.0711, 14.747) (31.8439, 14.747) (31.5508, 14.533) (31.4651, 14.3189) knots 0 0 0 1 2 2 2
  spline S78 degree 2 poles (31.4651, 14.3189) (31.3828, 14.1114) (31.3235, 13.4791) (31.3235, 13.0806) knots 0 0 0 1 2 2 2
  spline S79 degree 2 poles (31.3235, 13.0806) (31.3235, 12.6525) (31.3762, 12.0794) (31.4618, 11.8555) knots 0 0 0 1 2 2 2
  spline S80 degree 2 poles (31.4618, 11.8555) (31.5409, 11.6447) (31.834, 11.4175) (32.0711, 11.4175) knots 0 0 0 1 2 2 2
  spline S81 degree 2 poles (32.0711, 11.4175) (32.295, 11.4175) (32.5882, 11.6315) (32.6705, 11.8456) knots 0 0 0 1 2 2 2
  line L55 (36.3953, 11.0519) -> (33.889, 11.0519)
  line L56 (33.889, 11.0519) -> (33.889, 11.6282)
  spline S82 degree 2 poles (33.889, 11.6282) (34.1591, 11.8818) (34.6399, 12.3528) (34.8705, 12.6064) knots 0 0 0 1 2 2 2
  spline S83 degree 2 poles (34.8705, 12.6064) (35.3348, 13.1168) (35.674, 13.7294) (35.674, 14.0554) knots 0 0 0 1 2 2 2
  spline S84 degree 2 poles (35.674, 14.0554) (35.674, 14.2267) (35.5686, 14.4836) (35.4731, 14.5659) knots 0 0 0 1 2 2 2
  spline S85 degree 2 poles (35.4731, 14.5659) (35.3776, 14.6482) (35.1273, 14.7306) (34.9758, 14.7306) knots 0 0 0 1 2 2 2
  spline S86 degree 2 poles (34.9758, 14.7306) (34.8309, 14.7306) (34.5345, 14.6581) (34.3995, 14.6021) knots 0 0 0 1 2 2 2
  spline S87 degree 2 poles (34.3995, 14.6021) (34.2842, 14.556) (34.0702, 14.4243) (34.0043, 14.3782) knots 0 0 0 1 2 2 2
  line L57 (34.0043, 14.3782) -> (33.9747, 14.3782)
  line L58 (33.9747, 14.3782) -> (33.9747, 14.9578)
  spline S88 degree 2 poles (33.9747, 14.9578) (34.1426, 15.0402) (34.7453, 15.2015) (35.0154, 15.2015) knots 0 0 0 1 2 2 2
  spline S89 degree 2 poles (35.0154, 15.2015) (35.5851, 15.2015) (36.2273, 14.5988) (36.2273, 14.0851) knots 0 0 0 1 2 2 2
  spline S90 degree 2 poles (36.2273, 14.0851) (36.2273, 13.8447) (36.1153, 13.4429) (36.0165, 13.2716) knots 0 0 0 1 2 2 2
  spline S91 degree 2 poles (36.0165, 13.2716) (35.9177, 13.0938) (35.6312, 12.7447) (35.4731, 12.5767) knots 0 0 0 1 2 2 2
  spline S92 degree 2 poles (35.4731, 12.5767) (35.2163, 12.2968) (34.5872, 11.6974) (34.3995, 11.5228) knots 0 0 0 1 2 2 2
  line L59 (34.3995, 11.5228) -> (36.3953, 11.5228)
  line L60 (36.3953, 11.5228) -> (36.3953, 11.0519)
  spline S93 degree 2 poles (12.2846, 7.1796) (12.2846, 6.9162) (12.0969, 6.4419) (11.9289, 6.2773) knots 0 0 0 1 2 2 2
  spline S94 degree 2 poles (11.9289, 6.2773) (11.7182, 6.0698) (11.1484, 5.8557) (10.7137, 5.8557) knots 0 0 0 1 2 2 2
  line L61 (10.7137, 5.8557) -> (10.2559, 5.8557)
  line L62 (10.2559, 5.8557) -> (10.2559, 4.3408)
  line L63 (10.2559, 4.3408) -> (9.7158, 4.3408)
  line L64 (9.7158, 4.3408) -> (9.7158, 8.4048)
  line L65 (9.7158, 8.4048) -> (10.7367, 8.4048)
  spline S95 degree 2 poles (10.7367, 8.4048) (11.099, 8.4048) (11.6062, 8.2862) (11.8005, 8.1512) knots 0 0 0 1 2 2 2
  spline S96 degree 2 poles (11.8005, 8.1512) (12.0277, 7.9964) (12.2846, 7.5189) (12.2846, 7.1796) knots 0 0 0 1 2 2 2
  spline S97 degree 2 poles (11.7215, 7.1632) (11.7215, 7.374) (11.5766, 7.6835) (11.4284, 7.7823) knots 0 0 0 1 2 2 2
  spline S98 degree 2 poles (11.4284, 7.7823) (11.2999, 7.868) (10.9574, 7.9371) (10.7038, 7.9371) knots 0 0 0 1 2 2 2
  line L66 (10.7038, 7.9371) -> (10.2559, 7.9371)
  line L67 (10.2559, 7.9371) -> (10.2559, 6.3168)
  line L68 (10.2559, 6.3168) -> (10.6248, 6.3168)
  spline S99 degree 2 poles (10.6248, 6.3168) (10.9541, 6.3168) (11.3592, 6.4222) (11.4909, 6.5605) knots 0 0 0 1 2 2 2
  spline S100 degree 2 poles (11.4909, 6.5605) (11.6128, 6.6824) (11.7215, 6.9689) (11.7215, 7.1632) knots 0 0 0 1 2 2 2
  line L69 (14.3759, 6.8404) -> (14.3496, 6.8404)
  spline S101 degree 2 poles (14.3496, 6.8404) (14.2903, 6.8569) (14.1618, 6.8635) (14.0729, 6.8635) knots 0 0 0 1 2 2 2
  spline S102 degree 2 poles (14.0729, 6.8635) (13.8654, 6.8635) (13.4571, 6.6824) (13.2726, 6.5045) knots 0 0 0 1 2 2 2
  line L70 (13.2726, 6.5045) -> (13.2726, 4.3408)
  line L71 (13.2726, 4.3408) -> (12.7589, 4.3408)
  line L72 (12.7589, 4.3408) -> (12.7589, 7.3904)
  line L73 (12.7589, 7.3904) -> (13.2726, 7.3904)
  line L74 (13.2726, 7.3904) -> (13.2726, 6.9359)
  spline S103 degree 2 poles (13.2726, 6.9359) (13.5526, 7.1862) (13.9708, 7.3904) (14.1684, 7.3904) knots 0 0 0 1 2 2 2
  spline S104 degree 2 poles (14.1684, 7.3904) (14.2475, 7.3904) (14.3265, 7.3838) (14.3759, 7.374) knots 0 0 0 1 2 2 2
  line L75 (14.3759, 7.374) -> (14.3759, 6.8404)
  line L76 (15.298, 4.3408) -> (14.7843, 4.3408)
  line L77 (14.7843, 4.3408) -> (14.7843, 7.3904)
  line L78 (14.7843, 7.3904) -> (15.298, 7.3904)
  line L79 (15.298, 7.3904) -> (15.298, 4.3408)
  line L80 (15.3343, 7.8976) -> (14.7513, 7.8976)
  line L81 (14.7513, 7.8976) -> (14.7513, 8.4311)
  line L82 (14.7513, 8.4311) -> (15.3343, 8.4311)
  line L83 (15.3343, 8.4311) -> (15.3343, 7.8976)
  line L84 (18.4465, 4.3408) -> (17.9327, 4.3408)
  line L85 (17.9327, 4.3408) -> (17.9327, 6.0797)
  spline S105 degree 2 poles (17.9327, 6.0797) (17.9327, 6.2904) (17.8932, 6.6527) (17.8339, 6.7614) knots 0 0 0 1 2 2 2
  spline S106 degree 2 poles (17.8339, 6.7614) (17.7714, 6.8767) (17.5474, 6.9886) (17.3564, 6.9886) knots 0 0 0 1 2 2 2
  spline S107 degree 2 poles (17.3564, 6.9886) (17.1654, 6.9886) (16.7603, 6.7844) (16.566, 6.6198) knots 0 0 0 1 2 2 2
  line L86 (16.566, 6.6198) -> (16.566, 4.3408)
  line L87 (16.566, 4.3408) -> (16.0522, 4.3408)
  line L88 (16.0522, 4.3408) -> (16.0522, 7.3904)
  line L89 (16.0522, 7.3904) -> (16.566, 7.3904)
  line L90 (16.566, 7.3904) -> (16.566, 7.0512)
  spline S108 degree 2 poles (16.566, 7.0512) (16.7965, 7.2587) (17.2411, 7.476) (17.4914, 7.476) knots 0 0 0 1 2 2 2
  spline S109 degree 2 poles (17.4914, 7.476) (17.9393, 7.476) (18.4465, 6.8832) (18.4465, 6.3201) knots 0 0 0 1 2 2 2
  line L91 (18.4465, 6.3201) -> (18.4465, 4.3408)
  spline S110 degree 2 poles (20.0899, 4.2815) (19.6716, 4.2815) (19.2007, 4.759) (19.2007, 5.2761) knots 0 0 0 1 2 2 2
  line L92 (19.2007, 5.2761) -> (19.2007, 6.9656)
  line L93 (19.2007, 6.9656) -> (18.8549, 6.9656)
  line L94 (18.8549, 6.9656) -> (18.8549, 7.3904)
  line L95 (18.8549, 7.3904) -> (19.2007, 7.3904)
  line L96 (19.2007, 7.3904) -> (19.2007, 8.2665)
  line L97 (19.2007, 8.2665) -> (19.7144, 8.2665)
  line L98 (19.7144, 8.2665) -> (19.7144, 7.3904)
  line L99 (19.7144, 7.3904) -> (20.6596, 7.3904)
  line L100 (20.6596, 7.3904) -> (20.6596, 6.9656)
  line L101 (20.6596, 6.9656) -> (19.7144, 6.9656)
  line L102 (19.7144, 6.9656) -> (19.7144, 5.5132)
  spline S111 degree 2 poles (19.7144, 5.5132) (19.7144, 5.2827) (19.7309, 5.0291) (19.7869, 4.9204) knots 0 0 0 1 2 2 2
  spline S112 degree 2 poles (19.7869, 4.9204) (19.833, 4.8249) (20.0405, 4.7294) (20.2183, 4.7294) knots 0 0 0 1 2 2 2
  spline S113 degree 2 poles (20.2183, 4.7294) (20.3435, 4.7294) (20.5773, 4.8051) (20.63, 4.8282) knots 0 0 0 1 2 2 2
  line L103 (20.63, 4.8282) -> (20.6596, 4.8282)
  line L104 (20.6596, 4.8282) -> (20.6596, 4.3671)
  spline S114 degree 2 poles (20.6596, 4.3671) (20.5147, 4.3276) (20.2183, 4.2815) (20.0899, 4.2815) knots 0 0 0 1 2 2 2
  line L105 (25.7709, 8.4048) -> (24.3712, 4.3408)
  line L106 (24.3712, 4.3408) -> (23.7883, 4.3408)
  line L107 (23.7883, 4.3408) -> (22.3886, 8.4048)
  line L108 (22.3886, 8.4048) -> (22.9683, 8.4048)
  line L109 (22.9683, 8.4048) -> (24.0946, 5.0291)
  line L110 (24.0946, 5.0291) -> (25.2209, 8.4048)
  line L111 (25.2209, 8.4048) -> (25.7709, 8.4048)
  line L112 (27.579, 5.8722) -> (26.041, 5.8722)
  line L113 (26.041, 5.8722) -> (26.041, 6.3662)
  line L114 (26.041, 6.3662) -> (27.579, 6.3662)
  line L115 (27.579, 6.3662) -> (27.579, 5.8722)
  spline S115 degree 2 poles (30.6484, 6.3728) (30.6484, 5.2794) (30.0128, 4.2551) (29.3508, 4.2551) knots 0 0 0 1 2 2 2
  spline S116 degree 2 poles (29.3508, 4.2551) (28.6789, 4.2551) (28.0499, 5.2991) (28.0499, 6.3695) knots 0 0 0 1 2 2 2
  spline S117 degree 2 poles (28.0499, 6.3695) (28.0499, 7.4695) (28.6855, 8.4871) (29.3508, 8.4871) knots 0 0 0 1 2 2 2
  spline S118 degree 2 poles (29.3508, 8.4871) (30.0193, 8.4871) (30.6484, 7.4332) (30.6484, 6.3728) knots 0 0 0 1 2 2 2
  spline S119 degree 2 poles (29.9502, 5.1345) (30.0292, 5.3354) (30.0951, 5.9545) (30.0951, 6.3728) knots 0 0 0 1 2 2 2
  spline S120 degree 2 poles (30.0951, 6.3728) (30.0951, 6.791) (30.0292, 7.4069) (29.9469, 7.6144) knots 0 0 0 1 2 2 2
  spline S121 degree 2 poles (29.9469, 7.6144) (29.8646, 7.8219) (29.578, 8.0359) (29.3508, 8.0359) knots 0 0 0 1 2 2 2
  spline S122 degree 2 poles (29.3508, 8.0359) (29.1235, 8.0359) (28.8304, 7.8219) (28.7448, 7.6078) knots 0 0 0 1 2 2 2
  spline S123 degree 2 poles (28.7448, 7.6078) (28.6625, 7.4003) (28.6032, 6.768) (28.6032, 6.3695) knots 0 0 0 1 2 2 2
  spline S124 degree 2 poles (28.6032, 6.3695) (28.6032, 5.9413) (28.6559, 5.3683) (28.7415, 5.1444) knots 0 0 0 1 2 2 2
  spline S125 degree 2 poles (28.7415, 5.1444) (28.8206, 4.9336) (29.1137, 4.7063) (29.3508, 4.7063) knots 0 0 0 1 2 2 2
  spline S126 degree 2 poles (29.3508, 4.7063) (29.5747, 4.7063) (29.8678, 4.9204) (29.9502, 5.1345) knots 0 0 0 1 2 2 2
  line L116 (33.675, 4.3408) -> (31.1687, 4.3408)
  line L117 (31.1687, 4.3408) -> (31.1687, 4.9171)
  spline S127 degree 2 poles (31.1687, 4.9171) (31.4388, 5.1707) (31.9196, 5.6417) (32.1501, 5.8952) knots 0 0 0 1 2 2 2
  spline S128 degree 2 poles (32.1501, 5.8952) (32.6145, 6.4057) (32.9537, 7.0183) (32.9537, 7.3443) knots 0 0 0 1 2 2 2
  spline S129 degree 2 poles (32.9537, 7.3443) (32.9537, 7.5156) (32.8483, 7.7725) (32.7528, 7.8548) knots 0 0 0 1 2 2 2
  spline S130 degree 2 poles (32.7528, 7.8548) (32.6573, 7.9371) (32.407, 8.0195) (32.2555, 8.0195) knots 0 0 0 1 2 2 2
  spline S131 degree 2 poles (32.2555, 8.0195) (32.1106, 8.0195) (31.8142, 7.947) (31.6792, 7.891) knots 0 0 0 1 2 2 2
  spline S132 degree 2 poles (31.6792, 7.891) (31.5639, 7.8449) (31.3499, 7.7132) (31.284, 7.6671) knots 0 0 0 1 2 2 2
  line L118 (31.284, 7.6671) -> (31.2544, 7.6671)
  line L119 (31.2544, 7.6671) -> (31.2544, 8.2467)
  spline S133 degree 2 poles (31.2544, 8.2467) (31.4223, 8.329) (32.025, 8.4904) (32.2951, 8.4904) knots 0 0 0 1 2 2 2
  spline S134 degree 2 poles (32.2951, 8.4904) (32.8648, 8.4904) (33.507, 7.8877) (33.507, 7.374) knots 0 0 0 1 2 2 2
  spline S135 degree 2 poles (33.507, 7.374) (33.507, 7.1335) (33.395, 6.7318) (33.2962, 6.5605) knots 0 0 0 1 2 2 2
  spline S136 degree 2 poles (33.2962, 6.5605) (33.1974, 6.3827) (32.9109, 6.0336) (32.7528, 5.8656) knots 0 0 0 1 2 2 2
  spline S137 degree 2 poles (32.7528, 5.8656) (32.4959, 5.5857) (31.8669, 4.9863) (31.6792, 4.8117) knots 0 0 0 1 2 2 2
  line L120 (31.6792, 4.8117) -> (33.675, 4.8117)
  line L121 (33.675, 4.8117) -> (33.675, 4.3408)
  constraints: 4 end point, 2 midpoint, 1 horizontal, 1 perpendicular, 1 point on line
extrude "Extrusion12" cut sketch "Sketch12" against normal blind 1.27
split "Split6" plane through (0, 0, 0) removes the side toward (0, 0, 1)
equation "\"partDepth\" = 20.32"
equation "\"partWidth\" = 86.36"
body "Solid2"
